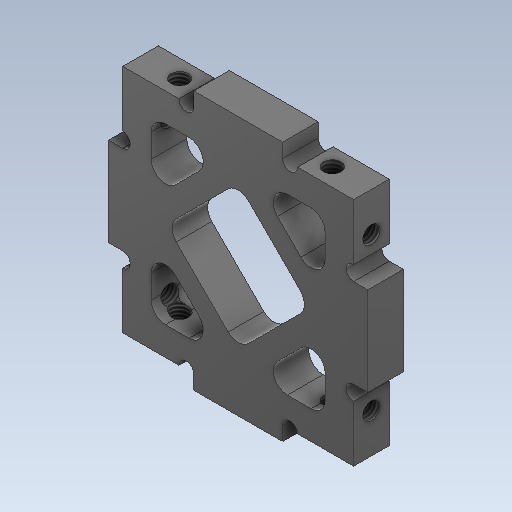
# Autodesk Inventor part: UpperArm_horizontal_frame_01
Saved by Autodesk Inventor 2020.4 (Build 244396000, 396)
## iProperties
Created: 2021-09-07
Part Number: UpperArm_horizontal_frame_01
Material: 一般
Document SubType Name: Modeling
Designer: aibay
Density: 1 g/cm^3
Appearance: 滑らか - 黒
Description: POM T5
Author: aibay
Autodesk Inventor part; units mm, degrees
ref_plane "YZ Plane" through (0, 0, 0) normal (1, 0, 0) x (0, 1, 0)
ref_plane "XZ Plane" through (0, 0, 0) normal (0, 1, 0) x (-1, 0, 0)
ref_plane "XY Plane" through (0, 0, 0) normal (0, 0, 1) x (1, 0, 0)
sketch "スケッチ1" plane through (0, 0, 0) normal (0, 0, 1) x (1, 0, 0)
  line L0 (0, 0) -> (16.25, 0)
  line L1 (16.25, 0) -> (16.25, 16.25)
  line L2 (16.25, 16.25) -> (0, 16.25)
  line L3 (0, 16.25) -> (0, 0)
  line L4 (16.25, 0) -> (8.95, 0)
  line L5 (0, 8.95) -> (0, 16.25)
  circle A0 centre (0, 8.95) radius 1.05
  circle A1 centre (8.95, 0) radius 1.05
  line L6 (16.25, 0) -> (10, 0)
  line L7 (10, 0) -> (10, -2)
  line L8 (10, -2) -> (16.25, -2)
  line L9 (16.25, -2) -> (16.25, 0)
  line L10 (0, 16.25) -> (-2, 16.25)
  line L11 (-2, 16.25) -> (-2, 10)
  line L12 (-2, 10) -> (0, 10)
  line L13 (0, 10) -> (0, 16.25)
  line L14 (6, 4) -> (9.3216, 4)
  line L15 (16.25, 4) -> (16.25, 16.25)
  line L16 (16.25, 16.25) -> (4, 16.25)
  line L17 (4, 9.3216) -> (4, 6)
  line L18 (7.4142, 10.7358) -> (10.7358, 7.4142)
  line L19 (6.1, 16.25) -> (0, 16.25)
  line L20 (7.5142, 14.8358) -> (14.8358, 7.5142)
  arc A2 (7.4142, 10.7358) -> (4, 9.3216) centre (6, 9.3216) ccw
  arc A3 (4, 6) -> (6, 4) centre (6, 6) ccw
  arc A4 (9.3216, 4) -> (10.7358, 7.4142) centre (9.3216, 6) ccw
  arc A5 (14.8358, 7.5142) -> (16.25, 6.9284) centre (16.25, 8.9284) ccw
  arc A6 (6.9284, 16.25) -> (7.5142, 14.8358) centre (8.9284, 16.25) ccw
  point P0 (4, 4)
  point P1 (4, 14.15)
  point P2 (16.25, 6.1)
  point P3 (0, 10)
  point P4 (0, 7.9)
  point P5 (7.9, 0)
  point P6 (16.25, 6.9284)
  dimension "d0" = 16.25
  dimension "d6" = 2.1
  dimension "d7" = 2.1
  dimension "d8" = 2
  dimension "d9" = 2
  dimension "d11" = 10.15
  dimension "d12" = 6.1
  dimension "d13" = 2
  constraints: 42 end point, 10 point on circle, 8 horizontal, 8 parallel, 8 point on line, 7 centre point, 7 tangent, 4 perpendicular, 2 coincident, 2 equal radius, 2 vertical, 7 other
  measures "d0" distance of L2.end L1.end
  measures "d6" diameter of A0
  measures "d7" diameter of A1
  measures "d8" distance of L7.end L6.end
  measures "d9" distance of L12.end L11.end
  measures "d11" distance of point (4, 4) point (4, 14.15)
  measures "d12" distance of point (16.25, 6.1) L0.end
  measures "d13" radius of A2
extrude "押し出し1" add sketch "スケッチ1" along normal blind 5 contours A1 L0 L3 A0 L2 A6 L20 A5 L1 | L0 L9 L8 L7 | L12 L11 L10 L3
sketch "スケッチ2" plane through (0, 0, 0) normal (0, -1, 0) x (1, 0, 0)
  circle A0 centre (5.5, 2.5) radius 1.25
  point P0 (0, 0)
  dimension "d17" = 2.5
  constraints: 1 centre point
  measures "d17" diameter of A0
hole "穴1" at (5.5, 0, 2.5) direction (0, 1, 0) diameter 2.459 depth 6 thread size "M3x0.5" class "6H" standard "ISO Metric profile"
sketch "スケッチ3" plane through (0, 0, 0) normal (-1, 0, 0) x (0, 0, 1)
  circle A0 centre (2.5, 5.5) radius 1.25
  point P0 (0, 0)
  dimension "d25" = 2.5
  constraints: 1 centre point
  measures "d25" diameter of A0
hole "穴2" at (0, 5.5, 2.5) direction (1, 0, 0) diameter 2.459 depth 6 thread size "M3x0.5" class "6H" standard "ISO Metric profile"
mirror "ミラー1" about plane through (16.25, -2, 0) normal (1, 0, 0) of "押し出し1", "穴1", "穴2"
mirror "ミラー2" about plane through (25.5716, 16.25, 0) normal (0, 1, 0) of "押し出し1", "穴1", "穴2", "ミラー1"
